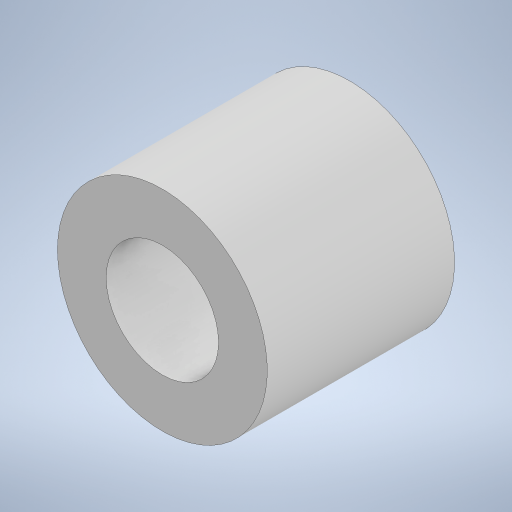
# Autodesk Inventor part: simple aperature
Saved by Autodesk Inventor 2024 (Build 280153000, 153)
## iProperties
Created: 2024-11-08
Part Number: simple aperature
Material: Generic
Document SubType Name: Modeling
Designer: Williamow
Density: 1 g/cm^3
Appearance: Default
Author: Williamow
Autodesk Inventor part; units mm, degrees
ref_plane "YZ Plane" through (0, 0, 0) normal (1, 0, 0) x (0, 1, 0)
ref_plane "XZ Plane" through (0, 0, 0) normal (0, 1, 0) x (-1, 0, 0)
ref_plane "XY Plane" through (0, 0, 0) normal (0, 0, 1) x (1, 0, 0)
sketch "Sketch1" plane through (0, 0, 0) normal (0, 1, 0) x (-1, 0, 0)
  line L0 (0, 0) -> (0, -4.4136)
  line L1 (2.8, 0) -> (2.8, -5)
  line L2 (2.8, -5) -> (0.25, -5)
  line L3 (0.25, -5) -> (0.25, -4.5)
  line L4 (0.25, -4.5) -> (1.5, -3.25)
  line L5 (1.5, -3.25) -> (1.5, 0)
  line L6 (1.5, 0) -> (2.8, 0)
  dimension "d0" = 2.8
  dimension "d1" = 1.5
  dimension "d2" = 5
  dimension "d3" = 0.5
  dimension "d4" = 135
  dimension "d5" = 0.25
  constraints: 14 end point, 3 perpendicular, 2 vertical, 1 horizontal alignment, 1 parallel
  measures "d0" distance of L0.start L1.start
  measures "d1" distance of L0.start L5.end
  measures "d2" distance of L1.start L1.end
  measures "d3" distance of L2.end L3.end
  measures "d4" angle of L3 L4
  measures "d5" distance between parallel lines of L0 L3
revolve "Revolution1" add sketch "Sketch1" angle 360 about axis through (0, 0, 0) along (0, 0, -1)
body "Solid1"
